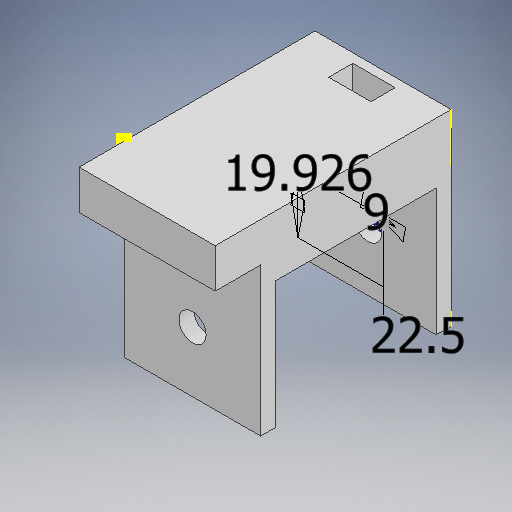
# Autodesk Inventor part: camera_case_bottom_new_left
Saved by Autodesk Inventor 2025.2 (Build 292293000, 293)
## iProperties
Created: 2025-03-10
Part Number: camera_case_bottom_new_left
Material: 일반
Document SubType Name: Modeling
Designer: jbhma
Density: 1 g/cm^3
Appearance: 기본값
Author: jbhma
Autodesk Inventor part; units mm, degrees
ref_plane "YZ Plane" through (0, 0, 0) normal (1, 0, 0) x (0, 1, 0)
ref_plane "XZ Plane" through (0, 0, 0) normal (0, 1, 0) x (-1, 0, 0)
ref_plane "XY Plane" through (0, 0, 0) normal (0, 0, 1) x (1, 0, 0)
sketch "스케치17" plane through (0, 0, 0) normal (1, 0, 0) x (0, 1, 0)
  line L0 (0, 0) -> (42, 0)
  line L1 (42, 0) -> (42, -5)
  line L2 (42, -5) -> (0, -5)
  line L3 (0, -5) -> (0, 0)
  line L4 (42, 0) -> (62, 0)
  line L5 (62, 0) -> (62, -63)
  line L6 (62, -63) -> (42, -63)
  line L7 (42, -63) -> (42, 0)
  line L8 (42, -63) -> (0, -63)
  line L9 (0, -63) -> (0, -58)
  line L10 (0, -58) -> (42, -58)
  line L11 (42, -58) -> (42, -63)
  dimension "d51" = 42
  dimension "d52" = 5
  dimension "d53" = 20
  dimension "d54" = 63
  dimension "d55" = 42
  dimension "d56" = 5
  constraints: 24 end point, 6 parallel, 3 horizontal, 3 perpendicular
  measures "d51" distance of L1.end L2.end
  measures "d52" distance of L0.end L1.end
  measures "d53" distance of L5.end L6.end
  measures "d54" distance of L4.end L5.end
  measures "d55" distance of L9.end L10.end
  measures "d56" distance of L8.end L9.end
extrude "돌출13" add sketch "스케치17" along normal blind 45
sketch "스케치18" plane through (0, 0, 0) normal (0, 0, 1) x (1, 0, 0)
  circle A0 centre (22.5, 19.926) radius 4.5
  line L0 (0, 0) -> (45, 0) projected
  line L1 (0, 62) -> (0, 0) projected
  dimension "d59" = 9
  dimension "d60" = 19.926
  dimension "d64" = 22.5
  constraints: 1 centre point
  measures "d59" diameter of A0
  measures "d60" distance from line of L0 A0.centre
  measures "d64" distance from line of A0.centre L1
sketch "스케치19" plane through (0, 0, -63) normal (0, 0, -1) x (-1, 0, 0)
  circle A0 centre (-22.5, 19.926) radius 4.5
  line L0 (0, 0) -> (-45, 0) projected
  line L1 (-45, 0) -> (-45, 62) projected
  point P0 (-22.5, 0)
  dimension "d61" = 9
  dimension "d62" = 19.926
  dimension "d63" = 22.5
  constraints: 1 centre point, 1 midpoint
  measures "d61" diameter of A0
  measures "d62" distance of A0.centre point (-22.5, 0)
  measures "d63" distance from line of A0.centre L1
extrude "돌출14" cut sketch "스케치18" against normal blind 100
sketch "스케치20" plane through (0, 62, 0) normal (0, 1, 0) x (1, 0, 0)
  point P0 (0, 0)
sketch "스케치21" plane through (0, 62, 0) normal (0, 1, 0) x (1, 0, 0)
  line L0 (15.5, 60) -> (29.5, 60)
  line L1 (29.5, 60) -> (29.5, 52)
  line L2 (29.5, 52) -> (15.5, 52)
  line L3 (15.5, 52) -> (15.5, 60)
  line L4 (0, 63) -> (0, 0) projected
  line L5 (0, 63) -> (45, 63) projected
  point P0 (15.5, 56)
  point P1 (22.5, 60)
  dimension "d67" = 14
  dimension "d68" = 8
  dimension "d69" = 15.5
  dimension "d70" = 3
  constraints: 8 end point, 2 midpoint, 2 parallel, 1 horizontal, 1 perpendicular
  measures "d67" distance of L1.end L2.end
  measures "d68" distance of L0.end L1.end
  measures "d69" distance from line of point (15.5, 56) L4
  measures "d70" distance from line of point (22.5, 60) L5
extrude "돌출15" cut sketch "스케치21" against normal blind 13
sketch "스케치27" plane through (0, 0, 0) normal (0, 0, 1) x (1, 0, 0)
  line L0 (0, 62) -> (45, 62)
  line L1 (45, 62) -> (45, 49)
  line L2 (45, 49) -> (0, 49)
  line L3 (0, 49) -> (0, 62)
  point P0 (0, 0)
  constraints: 8 end point, 2 parallel, 1 horizontal, 1 perpendicular
extrude "돌출21" add sketch "스케치27" along normal blind 15
